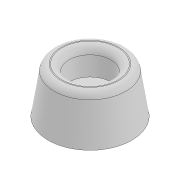
# Autodesk Inventor part: FOOT
Saved by Autodesk Inventor 2020 (Build 240168000, 168)
## iProperties
Created: 2020-04-13
Part Number: FOOT
Material: Generic
Document SubType Name: Modeling
Designer: John K
Density: 1 g/cm^3
Appearance: Default
Description: McM 9405K16
Author: John K
Autodesk Inventor part; units mm, degrees
ref_plane "YZ Plane" through (0, 0, 0) normal (1, 0, 0) x (0, 1, 0)
ref_plane "XZ Plane" through (0, 0, 0) normal (0, 1, 0) x (-1, 0, 0)
ref_plane "XY Plane" through (0, 0, 0) normal (0, 0, 1) x (1, 0, 0)
sketch "Sketch1" plane through (0, 0, 0) normal (0, 0, 1) x (1, 0, 0)
  line L0 (-1.9844, 4.3656) -> (-4.7625, 4.3656)
  line L1 (-4.7625, 4.3656) -> (-4.7625, 10.3188)
  line L2 (-4.7625, 10.3188) -> (-7.9375, 10.3187)
  line L3 (-7.9375, 10.3187) -> (-9.525, 0)
  line L4 (-9.525, 0) -> (-1.9844, 0)
  line L5 (0, 0) -> (0, -4.1368)
  line L6 (-1.9844, 4.3656) -> (-1.9844, 0)
  dimension "d0" = 9.525
  dimension "d1" = 19.05
  dimension "d2" = 4.3656
  dimension "d3" = 3.9688
  dimension "d4" = 10.3187
  dimension "d5" = 3.175
  constraints: 14 end point, 3 perpendicular, 1 horizontal, 1 horizontal alignment, 1 parallel, 1 vertical
  measures "d0" diameter of L1 L5
  measures "d1" diameter of L3.end L5
  measures "d2" distance between parallel lines of L4 L0
  measures "d3" diameter of L6 L5
  measures "d4" distance between parallel lines of L2 L4
  measures "d5" distance of L1.end L2.end
revolve "Revolution1" add sketch "Sketch1" angle 360 about axis through (0, 0, 0) along (0, -1, 0)
fillet "Fillet1" radius 1.5875 2 edges at (7.9375, 10.3187, 0) (4.7625, 10.3188, 0)
body "Solid1"
